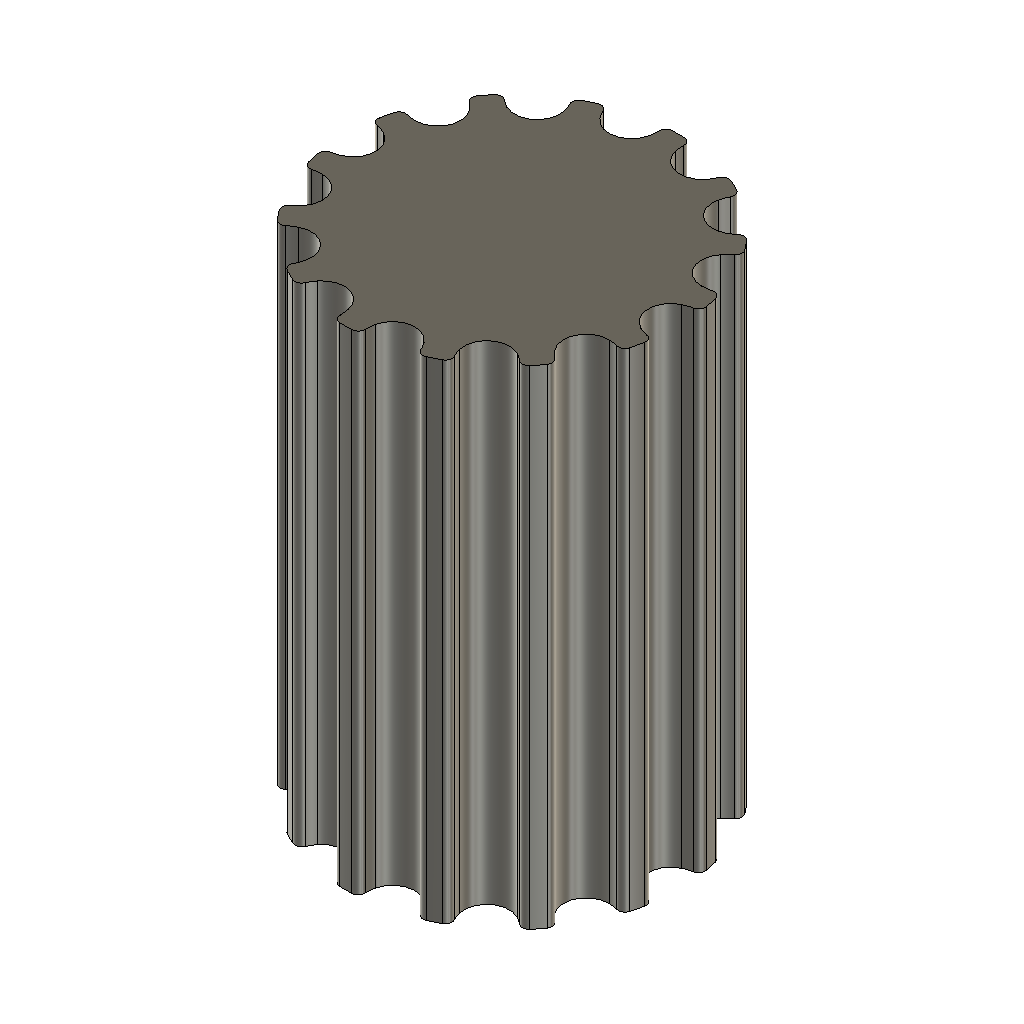
GT2-3M Generator (Autodesk Fusion 360 design; units mm, degrees)
Autodesk Fusion 360 part; units mm, degrees
sketch "Teeth" plane through (0, 0, 0) normal (0, 0, 1) x (1, 0, 0)
  circle A0 centre (0, 0) radius 6.6845
  arc A1 (0.5054, 5.6922) -> (1.149, 5.0341) centre (1.3381, 5.8627) ccw
  line L0 (0, 0) -> (0, 7.1835) construction
  line L1 (0, 0) -> (1.3381, 5.8627) construction
  line L2 (0, 6.3035) -> (0, 6.6845)
  arc A2 (1.4874, 6.5169) -> (0, 6.6845) centre (0, 0) ccw
  arc A3 (0.2346, 6.2991) -> (0, 6.3035) centre (0, 0) ccw
  arc A4 (0.4752, 6.042) -> (0.2346, 6.2991) centre (0.2253, 6.0493) ccw
  arc A5 (0.4752, 6.042) -> (0.5054, 5.6922) centre (1.9945, 5.9972) ccw
  line L3 (1.4874, 6.5169) -> (2.0822, 6.3812) construction
  line L4 (1.9945, 5.9972) -> (2.0822, 6.3812) construction
  arc A6 (1.149, 5.0341) -> (2.0144, 5.3478) centre (1.3381, 5.8627) ccw
  arc A7 (2.0144, 5.3478) -> (2.1934, 5.6498) centre (0.8051, 6.2687) ccw
  arc A8 (2.5218, 5.7771) -> (2.1934, 5.6498) centre (2.4217, 5.548) ccw
  arc A9 (2.735, 5.6793) -> (2.5218, 5.7771) centre (0, 0) ccw
  line L5 (2.735, 5.6793) -> (2.9003, 6.0225)
  arc A10 (2.9003, 6.0225) -> (1.4874, 6.5169) centre (0, 0) ccw
  dimension "d50" = 13.369
  dimension "d59" = 12.857
  dimension "d67" = 0.381
  dimension "d68" = 0.25
  dimension "d69" = 1.521
  dimension "d71" = 0.61
  dimension "d72" = 0.85
  dimension "d73" = 1.52
  constraint coincident A0.centre L0.start
  constraint coincident A0 L2.end
  constraint parallel L0 L2
  constraint coincident A0 A2.start
  constraint collinear A1.centre A0.centre A2.start
  constraint coincident A1.centre L1.end
  constraint coincident L1 A1.end
  constraint vertical L0
  constraint coincident L0 L2.start
  constraint tangent A3 A4
  constraint tangent A4 A5
  constraint tangent A1 A5
  constraint tangent A0 L3
  constraint coincident A5.centre L4.start
  constraint coincident L3 L4.end
  constraint perpendicular L3 L4
  constraint coincident L3.end L4.end
  constraint symmetric A1 L1 A6
  constraint symmetric L1 L2.end L5.end
  constraint symmetric L1 A2.start L3.start
  constraint symmetric L1 A2 A10
  constraint symmetric L1 A1.end A6.start
  constraint symmetric L1 L2.start A9.start
  constraint symmetric L1 A3.start A8.start
  constraint symmetric L1 A3 A9
  constraint symmetric L1 A4.start A7.end
  constraint symmetric L1 A4 A8
  constraint symmetric L1 A1.start A6.end
  constraint symmetric L1 A5 A7
  measures "d50" diameter of A0
  measures "d59" angle of L0 L1
  measures "d67" distance of L2.end L2.start
  measures "d68" radius of A4
  measures "d69" distance of A2.start A1.end
  measures "d71" distance of A2.start L3.end
  measures "d72" radius of A1
  measures "d73" radius of A5
extrude "Extrude1" add sketch "Teeth" along normal mid plane 18.5
extrude "Extrude3" cut sketch "Teeth" along normal through all and the other way through all contours A0 A1 L2 A2 A3 A4 A5 A6 A7 A8 A9 L5 A10
pattern_circular "C-Pattern1" count 14 over 360 about axis through (0, 0, 0) along (0, 0, 1) of "Extrude3"
equation "p = 3 mm"
equation "n = 14" comment "Number of Teeth"
equation "PD = n * p / 3.14159"
equation "d25 = width"
equation "d50 = PD"
equation "d52 = n"
equation "d59 = ( 180 / n ) * 1 deg"
equation "width = 18.5 mm"
